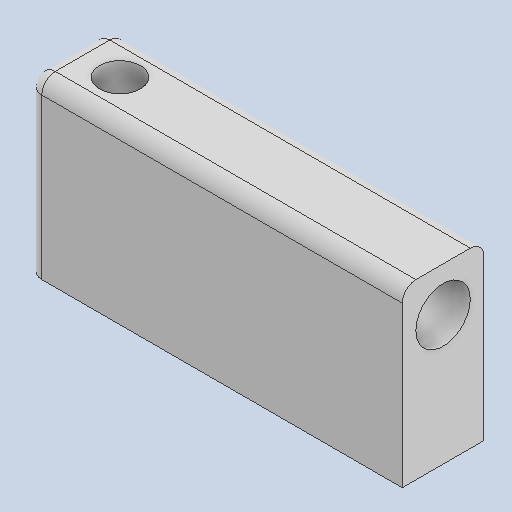
# Autodesk Inventor part: cilinder
Saved by Autodesk Inventor 2022.2 (Build 262287010, 287A)
## iProperties
Created: 2022-05-04
Part Number: cilinder
Material: Genérico
Document SubType Name: Modeling
Designer: 19710060
Density: 1 g/cm^3
Appearance: Padrão
Author: 19710060
Autodesk Inventor part; units mm, degrees
ref_plane "YZ Plane" through (0, 0, 0) normal (1, 0, 0) x (0, 1, 0)
ref_plane "XZ Plane" through (0, 0, 0) normal (0, 1, 0) x (-1, 0, 0)
ref_plane "XY Plane" through (0, 0, 0) normal (0, 0, 1) x (1, 0, 0)
sketch "Esboço2" plane through (0, 0, 0) normal (0, 1, 0) x (-1, 0, 0)
  line L0 (0, 0) -> (-55, 0)
  line L1 (-55, 0) -> (-55, -12)
  line L2 (-55, -12) -> (0, -12)
  line L3 (0, -12) -> (0, 0)
  dimension "d0" = 55
  dimension "d1" = 12
  constraints: 8 end point, 2 parallel, 1 horizontal, 1 perpendicular
  measures "d0" distance of L2.end L1.end
  measures "d1" distance of L1.end L0.end
extrude "Extrusão1" add sketch "Esboço2" along normal blind 25.5
sketch "Esboço3" plane through (0, 25.5, 0) normal (0, 1, 0) x (1, 0, 0)
  line L0 (0, 12) -> (0, 0) projected
  line L1 (0, 6) -> (7.5, 6)
  dimension "d4" = 7.5
  constraints: 2 end point, 1 coincident, 1 horizontal, 1 midpoint
  measures "d4" distance of L1.start L1.end
hole "Furo1" at (7.5, 25.5, -6) direction (0, -1, 0) diameter 6 end through all
sketch "Esboço4" plane through (0, 0, 0) normal (0, -1, 0) x (1, 0, 0)
  circle A0 centre (7.5, -6) radius 3 projected
  line L0 (7.5, -6) -> (20.7, -6)
  point P0 (0, 0)
  dimension "d12" = 13.2
  constraints: 2 end point, 1 horizontal
  measures "d12" distance of L0.start L0.end
sketch "Esboço5" plane through (55, 0, 0) normal (1, 0, 0) x (0, 0, -1)
  line L0 (0, 0) -> (0, 19)
  line L1 (0, 0) -> (0, 25.5) projected
  line L2 (0, 19) -> (6, 19)
  dimension "d13" = 19
  dimension "d14" = 6
  constraints: 4 end point, 1 perpendicular, 1 point on line
  measures "d13" distance of L0.start L0.end
  measures "d14" distance of L0.end L2.end
hole "Furo2" at (55, 19, -6) direction (-1, 0, 0) diameter 8 depth 41
hole "Furo3" at (20.7, 0, -6) direction (0, 1, 0) diameter 2 depth 16
fillet "Arredondamento1" radius 2 5 edges at (0, 25.5, -6) (0, 12.75, 0) (0, 12.75, -12) (27.5, 25.5, 0) (27.5, 25.5, -12)
